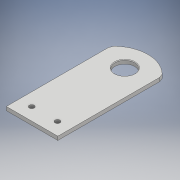
# Autodesk Inventor part: platen_support
Saved by Autodesk Inventor 2018 (Build 220112000, 112)
## iProperties
Created: 2018-10-27
Part Number: platen_support
Material: Generic
Document SubType Name: Modeling
Designer: Fredy Espana C
Density: 1 g/cm^3
Appearance: Default
Author: Fredy Espana C
Autodesk Inventor part; units mm, degrees
ref_plane "YZ Plane" through (0, 0, 0) normal (1, 0, 0) x (0, 1, 0)
ref_plane "XZ Plane" through (0, 0, 0) normal (0, 1, 0) x (-1, 0, 0)
ref_plane "XY Plane" through (0, 0, 0) normal (0, 0, 1) x (1, 0, 0)
sketch "Sketch2" plane through (0, 0, 0) normal (0, 0, 1) x (1, 0, 0)
  line L0 (0, 0) -> (44.45, 0)
  line L1 (44.45, 0) -> (44.45, 90)
  line L2 (0, 90) -> (0, 0)
  arc A0 (44.45, 90) -> (0, 90) centre (22.225, 70.3025) ccw
  dimension "d3" = 44.45
  dimension "d4" = 100
  dimension "d5" = 90
  constraints: 6 end point, 2 parallel, 2 point on circle, 1 centre point, 1 horizontal, 1 perpendicular
  measures "d3" distance of L0.start L0.end
  measures "d5" distance of L0.end L1.end
extrude "Extrusion1" add sketch "Sketch2" along normal blind 3.175
chamfer "Chamfer1" distance 2 angle 45 2 edges at (44.45, 90, 1.5875) (0, 90, 1.5875)
sketch "Sketch3" plane through (0, 0, 3.175) normal (0, 0, 1) x (1, 0, 0)
  line L0 (0, 88) -> (0, 0) projected
  line L1 (0, 0) -> (44.45, 0) projected
  point P0 (22.225, 80)
  point P1 (22.225, 0)
  dimension "d13" = 80
  constraints: 1 midpoint, 1 vertical alignment
  measures "d13" distance from line of L1 point (22.225, 80)
hole "Hole1" at (22.225, 80, 3.175) direction (0, 0, -1) diameter 17 end through all
fillet "Fillet1" radius 0.5 1 edges at (22.225, 88.5, 3.175)
sketch "Sketch4" plane through (0, 0, 3.175) normal (0, 0, 1) x (1, 0, 0)
  line L0 (0, 0) -> (44.45, 0) projected
  line L1 (0, 88) -> (0, 0) projected
  line L2 (44.45, 0) -> (44.45, 88) projected
  point P0 (11.1125, 10.7938)
  point P1 (33.325, 10.7938)
  dimension "d22" = 44.45
  dimension "d23" = 11.1125
  dimension "d24" = 11.125
  constraints: 1 horizontal alignment
  measures "d22" distance of L0.start L0.end
  measures "d23" distance from line of L1 point (11.113, 10.794)
  measures "d24" distance from line of L2 point (33.325, 10.794)
hole "Hole2" at (11.1125, 10.7938, 3.175) at (33.325, 10.7938, 3.175) direction (0, 0, -1) diameter 4.2333 end through all
body "Solid1"
